Autodesk Inventor part; units mm, degrees
(part 4 of 4)
sketch "スケッチ16" plane through (0, 0, 10) normal (0, 0, 1) x (1, 0, 0)
  line L0 (-0.25, -101.281) -> (8.75, -101.281) projected
  line L1 (-0.25, 101.281) -> (-0.25, -101.281) projected
  point P0 (0, 0)
  point P1 (4.25, -91.281)
  point P2 (4.25, -51.281)
  point P3 (4.25, -11.281)
  point P4 (4.25, 90.719)
  dimension "d78" = 10
  dimension "d79" = 4.5
  dimension "d80" = 40
  dimension "d81" = 40
  dimension "d82" = 102
  dimension "d83" = 4.5
  measures "d78" distance from line of L0 point (4.25, -91.281)
  measures "d79" distance from line of L1 point (4.25, -91.281)
  measures "d80" distance of point (4.25, -91.281) point (4.25, -51.281)
  measures "d81" distance of point (4.25, -11.281) point (4.25, -51.281)
  measures "d82" distance of point (4.25, 90.719) point (4.25, -11.281)
  measures "d83" distance from line of L1 point (4.25, 90.719)
hole "穴3" at (4.25, -91.281, 10) at (4.25, -51.281, 10) at (4.25, -11.281, 10) at (4.25, 90.719, 10) direction (0, 0, -1) diameter 3.2 end through all
